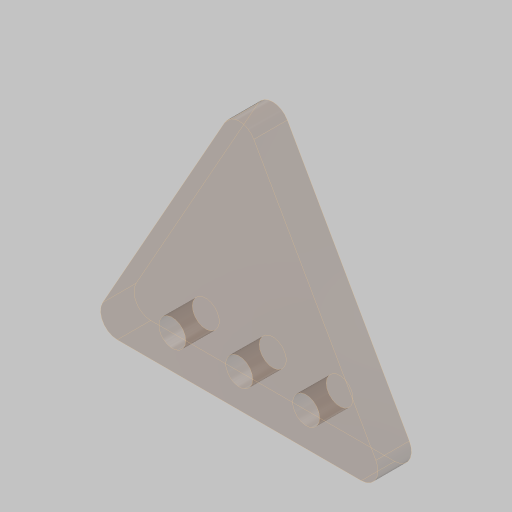
# Autodesk Inventor part: CL7-017
Saved by Autodesk Inventor 2023.5 (Build 275446000, 446)
## iProperties
Created: 2025-03-19
Part Number: CL7-017
Material: Polycarbonate, Smoke
Document SubType Name: Modeling
Designer: slick
Density: 1.2 g/cm^3
Appearance: Polycarbonate - Smoked
Author: slick
Autodesk Inventor part; units mm, degrees
ref_plane "YZ Plane" through (0, 0, 0) normal (1, 0, 0) x (0, 1, 0)
ref_plane "XZ Plane" through (0, 0, 0) normal (0, 1, 0) x (-1, 0, 0)
ref_plane "XY Plane" through (0, 0, 0) normal (0, 0, 1) x (1, 0, 0)
sketch "Sketch1" plane through (0, 0, 0) normal (0, 0, 1) x (1, 0, 0)
  line L0 (28.575, 0) -> (-28.575, 0)
  line L1 (-28.575, 0) -> (0, 50.8)
  line L2 (0, 50.8) -> (28.575, 0)
  point P0 (0, 0)
  point P1 (0, 0)
  dimension "d0" = 57.15
  dimension "d1" = 50.8
  constraints: 7 end point, 1 coincident, 1 equal length, 1 horizontal, 1 midpoint, 1 vertical alignment
  measures "d0" distance of L0.start L0.end
  measures "d1" distance from line of L0 L1.end
extrude "Extrusion1" add sketch "Sketch1" along normal blind 6.35
fillet "Fillet1" radius 3.175 3 edges at (28.575, 0, 3.175) (-28.575, 0, 3.175) (0, 50.8, 3.175)
sketch "Sketch2" plane through (0, 0, 6.35) normal (0, 0, 1) x (1, 0, 0)
  line L0 (-12.7, 6.35) -> (12.7, 6.35) construction
  line L1 (-23.1462, 0) -> (23.1462, 0) construction
  point P0 (0, 0)
  point P1 (0, 6.35)
  point P2 (0, 6.35)
  point P3 (0, 0)
  dimension "d5" = 6.35
  dimension "d6" = 25.4
  constraints: 2 end point, 2 horizontal alignment, 2 midpoint, 1 coincident, 1 horizontal, 1 vertical alignment
  measures "d5" distance between parallel lines of L1 L0
  measures "d6" distance of L0.start L0.end
hole "Hole1" at (-12.7, 6.35, 6.35) at (0, 6.35, 6.35) at (12.7, 6.35, 6.35) direction (0, 0, -1) diameter 5.1054 end through all start extended yes clearance for "Flat Head Machine Screw (82)" size "#10" standard "Ansi Unified Screw Threads"
body "Solid1"
